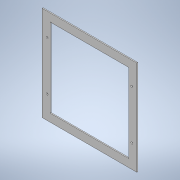
# Autodesk Inventor part: TurretBasePlate
Saved by Autodesk Inventor 2022 (Build 260153000, 153)
## iProperties
Created: 2022-01-15
Part Number: TurretBasePlate
Material: Generic
Document SubType Name: Modeling
Designer: Ty Gazaway
Density: 1 g/cm^3
Appearance: Default
Author: Ty Gazaway
Autodesk Inventor part; units mm, degrees
ref_plane "YZ Plane" through (0, 0, 0) normal (1, 0, 0) x (0, 1, 0)
ref_plane "XZ Plane" through (0, 0, 0) normal (0, 1, 0) x (-1, 0, 0)
ref_plane "XY Plane" through (0, 0, 0) normal (0, 0, 1) x (1, 0, 0)
sketch "Sketch1" plane through (0, 0, 0) normal (0, 0, 1) x (1, 0, 0)
  line L0 (0, 0) -> (304.8, 0)
  line L1 (304.8, 0) -> (304.8, 304.8)
  line L2 (304.8, 304.8) -> (0, 304.8)
  line L3 (0, 304.8) -> (0, 0)
  line L4 (25.4, 25.4) -> (279.4, 25.4)
  line L5 (279.4, 25.4) -> (279.4, 279.4)
  line L6 (279.4, 279.4) -> (25.4, 279.4)
  line L7 (25.4, 279.4) -> (25.4, 25.4)
  circle A0 centre (15.875, 231.15) radius 3.175
  circle A1 centre (288.673, 231.15) radius 3.175
  circle A2 centre (15.875, 73.65) radius 3.175
  circle A3 centre (288.673, 73.65) radius 3.175
  dimension "d0" = 304.8
  dimension "d1" = 304.8
  dimension "d2" = 254
  dimension "d3" = 254
  dimension "d4" = 25.4
  dimension "d5" = 25.4
  dimension "d8" = 6.35
  dimension "d9" = 73.65
  dimension "d10" = 15.875
  dimension "d13" = 272.798
  dimension "d16" = 157.5
  constraints: 16 end point, 4 centre point, 4 parallel, 3 horizontal, 2 perpendicular, 1 vertical, 6 other
  measures "d0" distance of L2.end L1.end
  measures "d1" distance of L1.end L0.end
  measures "d2" distance of L6.end L5.end
  measures "d3" distance of L5.end L4.end
  measures "d4" distance between parallel lines of L2 L6
  measures "d5" distance between parallel lines of L1 L5
  measures "d8" diameter of A0
  measures "d9" distance from line of L2 A0.centre
  measures "d10" distance from line of L3 A0.centre
  measures "d13" distance of A0.centre A1.centre
  measures "d16" distance of A0.centre A2.centre
extrude "Extrusion1" add sketch "Sketch1" along normal blind 3.175
body "Solid1"
